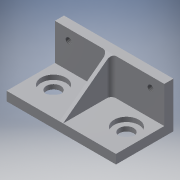
# Autodesk Inventor part: M178-3502
Saved by Autodesk Inventor 2018 (Build 220105000, 105)
## iProperties
Created: 2004-11-29
Part Number: M178-3502
Document SubType Name: Modeling
Designer: Autodesk, Inc.
Manufacturer: Standard
Standards Organization: Custom
Material: Aluminum-6061
Description: SWING ARM MOUNT BRACKET
Mass: 83.1425 g
Surface Area: 128.488 cm^2
Volume: 30.6799 cm^3
Density: 2.71 g/cm^3
Appearance: Aluminum - Flat
CAGE: 1LJX3
Dept. ID: Product Design
Description #2: ---
Finish #1: ---
Finish #2: ---
Material ID: ---
Project Number: ---
Author: Autodesk, Inc.
Autodesk Inventor part; units mm, degrees
ref_plane "YZ Plane" through (0, 0, 0) normal (1, 0, 0) x (0, 1, 0)
ref_plane "XZ Plane" through (0, 0, 0) normal (0, 1, 0) x (-1, 0, 0)
ref_plane "XY Plane" through (0, 0, 0) normal (0, 0, 1) x (1, 0, 0)
sketch "Sketch1" plane through (0, 0, 0) normal (0, 0, 1) x (1, 0, 0)
  line L0 (-20, 6.35) -> (20, 6.35)
  line L1 (20, 6.35) -> (20, 0)
  line L2 (20, 0) -> (-20, 0)
  line L3 (-20, 0) -> (-20, 6.35)
  line L4 (20, 0) -> (13.65, 0)
  line L5 (13.65, 0) -> (13.65, 31.75)
  line L6 (13.65, 31.75) -> (20, 31.75)
  line L7 (20, 31.75) -> (20, 0)
  point P0 (0, 0)
  point P1 (0, 0)
  dimension "d0" = 40
  dimension "d1" = 31.75
  dimension "d2" = 6.35
  constraints: 16 end point, 4 parallel, 3 perpendicular, 2 horizontal, 2 midpoint, 1 coincident
  measures "d0" distance of L1.end L2.end
  measures "d1" distance of L6.end L1.end
  measures "d2" distance of L5.end L6.end
extrude "Extrusion1" add sketch "Sketch1" along normal mid plane 76.2
sketch "Sketch2" plane through (13.65, 31.75, 38.1) normal (0, 1, 0) x (1, 0, 0)
  line L0 (-33.65, 0) -> (-33.65, 76.2) projected
  line L1 (0, 76.2) -> (0, 0) projected
  line L2 (0, 38.1) -> (-33.65, 38.1)
  constraints: 2 end point, 2 midpoint
rib "Rib1" sketch "Sketch2" thickness 2.54 direction (0, -1, 0) end up to next extend profile no curves L2
sketch "Sketch3" plane through (-20, 31.75, 1.27) normal (0, 0, 1) x (1, 0, 0)
  line L0 (33.65, -25.4) -> (0, -25.4) projected
  line L1 (33.65, 0) -> (33.65, -25.4) projected
  line L2 (0, 0) -> (33.65, 0) projected
  line L3 (0, 0) -> (0, -25.4) projected
  line L4 (0, -25.4) -> (33.65, 0)
  constraints: 2 end point
extrude "Extrusion2" cut sketch "Sketch3" against normal through all contours L3 L2 L4
fillet "Fillet1" radius 3.175 2 edges at (13.65, 19.05, 1.27) (13.65, 19.05, -1.27)
sketch "Sketch4" plane through (-20, 6.35, 38.1) normal (0, 1, 0) x (1, 0, 0)
  line L0 (0, 0) -> (0, 36.83) projected
  line L1 (0, 0) -> (33.65, 0) projected
  point P0 (20, 12.7)
  dimension "d10" = 20
  dimension "d11" = 12.7
  measures "d10" distance from line of point (20, 12.7) L0
  measures "d11" distance from line of L1 point (20, 12.7)
hole "Hole1" at (0, 6.35, 25.4) direction (0, -1, 0) diameter 10.0076 end through all counterbore diameter 17.272 counterbore depth 3.175
mirror "Mirror1" about plane through (0, 0, 0) normal (0, 0, 1) of "Hole1"
sketch "Sketch5" plane through (13.65, 6.35, 38.1) normal (-1, 0, 0) x (0, 0, 1)
  circle A0 centre (-9.525, 18.1) radius 2.54
  constraints: 1 centre point, 1 other
hole "Hole2" at (13.65, 24.45, 28.575) direction (1, 0, 0) diameter 4.1402 end through all
mirror "Mirror2" about plane through (0, 0, 0) normal (0, 0, 1) of "Hole2"
body "Solid1"
